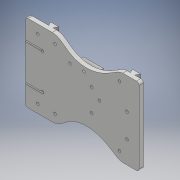
# Autodesk Inventor part: one_part_body_V2
Saved by Autodesk Inventor 2017 (Build 210142000, 142)
## iProperties
Created: 2017-05-19
Part Number: one_part_body_V2
Material: Generic
Document SubType Name: Modeling
Designer: Andi
Density: 1 g/cm^3
Appearance: Default
Author: Andi
Autodesk Inventor part; units mm, degrees
ref_plane "YZ Plane" through (0, 0, 0) normal (1, 0, 0) x (0, 1, 0)
ref_plane "XZ Plane" through (0, 0, 0) normal (0, 1, 0) x (-1, 0, 0)
ref_plane "XY Plane" through (0, 0, 0) normal (0, 0, 1) x (1, 0, 0)
sketch "Sketch1" plane through (0, 0, 0) normal (0, 1, 0) x (-1, 0, 0)
  line L0 (0, 90) -> (-132, 90)
  line L1 (-132, 90) -> (-132, 0)
  line L2 (-132, 0) -> (0, 0)
  line L3 (0, 0) -> (0, 90)
  line L4 (0, 45) -> (-132, 45)
  line L5 (0, 65.5) -> (-20, 65.5)
  line L6 (-20, 65.5) -> (-20, 67)
  line L7 (-20, 67) -> (0, 67)
  line L8 (0, 67) -> (0, 65.5)
  line L9 (0, 23) -> (-20, 23)
  line L10 (-20, 23) -> (-20, 24.5)
  line L11 (-20, 24.5) -> (0, 24.5)
  line L12 (0, 24.5) -> (0, 23)
  circle A0 centre (-20, 65.5) radius 1.5
  circle A1 centre (-20, 24.5) radius 1.5
  dimension "d0" = 132
  dimension "d1" = 90
  dimension "d2" = 20
  dimension "d3" = 41
  dimension "d4" = 1.5
  dimension "d5" = 1.5
  constraints: 26 end point, 6 parallel, 3 coincident, 3 horizontal, 3 perpendicular, 3 point on line, 2 midpoint, 2 vertical alignment, 1 symmetric about line, 4 other
  measures "d0" distance of L2.end L1.end
  measures "d1" distance of L2.end L0.start
  measures "d2" distance of L6.end L7.end
  measures "d3" distance of L11.end L5.start
  measures "d4" distance of L5.end L6.end
  measures "d5" distance of L9.end L10.end
extrude "Extrusion1" add sketch "Sketch1" along normal blind 5 contours L3 L7 A0 L5 L4 L1 L0 | L4 L3 L11 A1 L9 L2 L1
sketch "Sketch2" plane through (0, 0, 90) normal (0, 0, 1) x (1, 0, 0)
  line L0 (0, 5) -> (132, 5) projected
  line L1 (22, 5) -> (19.75, 9.5)
  line L2 (19.75, 9.5) -> (29.25, 9.5)
  line L3 (29.25, 9.5) -> (27, 5)
  line L4 (24.5, 9.5) -> (24.5, 0)
  line L5 (132, 0) -> (0, 0) projected
  line L6 (72, 0) -> (72, 13)
  line L7 (132, 0) -> (132, 5) projected
  line L8 (122, 5) -> (124.25, 9.5)
  line L9 (124.25, 9.5) -> (114.75, 9.5)
  line L10 (114.75, 9.5) -> (117, 5)
  line L11 (117, 5) -> (122, 5)
  line L12 (132, 5) -> (0, 5) projected
  dimension "d8" = 9.5
  dimension "d10" = 22
  dimension "d11" = 5
  dimension "d15" = 4.5
  dimension "d90" = 60
  constraints: 18 end point, 4 point on line, 4 symmetric about line, 2 perpendicular, 1 collinear, 1 midpoint, 1 parallel, 1 vertical, 1 other
  measures "d8" distance of L1.end L2.end
  measures "d10" distance of L1.start L0.start
  measures "d11" distance of L3.end L1.start
  measures "d15" distance between parallel lines of L2 L0
  measures "d90" distance between parallel lines of L7 L6
extrude "Extrusion7" add sketch "Sketch2" against normal up to surface (90 mm away) contours L10 L9 L8 L0 | L0 L4 L2 L3 | L0 L1 L2 L4
sketch "Sketch3" plane through (132, 0, 90) normal (1, 0, 0) x (0, 0, -1)
  line L0 (0, 0) -> (90, 0) projected
  line L1 (0, 9.5) -> (90, 9.5) projected
  line L2 (90, 5) -> (0, 5) projected
  line L3 (22.5, 9.5) -> (67.5, 9.5)
  line L4 (67.5, 9.5) -> (67.5, 5)
  line L5 (67.5, 5) -> (22.5, 5)
  line L6 (22.5, 5) -> (22.5, 9.5)
  line L7 (0, 9.5) -> (0, 5) projected
  line L8 (90, 5) -> (90, 9.5) projected
  dimension "d93" = 45
  dimension "d94" = 22.5
  dimension "d95" = 22.5
  constraints: 8 end point, 2 parallel, 2 point on line, 1 horizontal, 1 perpendicular
  measures "d93" distance between parallel lines of L4 L6
  measures "d94" distance between parallel lines of L7 L6
  measures "d95" distance between parallel lines of L8 L4
extrude "Extrusion3" cut sketch "Sketch3" against normal blind 120 contours L1 L4 L2 L6
sketch "Sketch4" plane through (0, 5, 0) normal (0, 1, 0) x (1, 0, 0)
  line L0 (50, -27) -> (70, -27)
  line L1 (70, -27) -> (70, -63)
  line L2 (70, -63) -> (50, -63)
  line L3 (50, -63) -> (50, -66)
  line L4 (50, -66) -> (73, -66)
  line L5 (73, -66) -> (73, -24)
  line L6 (73, -24) -> (50, -24)
  line L7 (50, -24) -> (50, -27)
  line L8 (132, -90) -> (132, 0) projected
  line L9 (132, -45) -> (0, -45)
  line L10 (0, -24.5) -> (0, -65.5) projected
  point P0 (0, 0)
  dimension "d25" = 3
  dimension "d26" = 70
  dimension "d27" = 3
  dimension "d28" = 20
  dimension "d29" = 36
  constraints: 18 end point, 7 perpendicular, 2 horizontal, 1 midpoint, 1 point on line, 2 other
  measures "d25" distance of L6.end L0.start
  measures "d26" distance between parallel lines of L10 L1
  measures "d27" distance between parallel lines of L1 L5
  measures "d28" distance of L0.start L0.end
  measures "d29" distance of L0.end L1.end
extrude "Extrusion4" add sketch "Sketch4" along normal blind 11
sketch "Sketch5" plane through (0, 16, 0) normal (0, 1, 0) x (1, 0, 0)
  line L0 (73, -24) -> (50, -24) projected
  line L1 (50, -63) -> (50, -66) projected
  line L2 (73, -24) -> (50, -24)
  line L3 (50, -24) -> (50, -66)
  line L4 (50, -66) -> (73, -66)
  line L5 (73, -66) -> (73, -24)
  point P0 (0, 0)
  constraints: 8 end point, 2 parallel, 1 horizontal, 1 perpendicular
extrude "Extrusion5" add sketch "Sketch5" along normal blind 2
sketch "Sketch6" plane through (0, 0, 0) normal (0, -1, 0) x (1, 0, 0)
  line L0 (67.1453, 53) -> (87.1453, 53)
  line L1 (87.1453, 53) -> (87.1453, 37)
  line L2 (87.1453, 37) -> (67.1453, 37)
  line L3 (67.1453, 37) -> (67.1453, 53)
  line L4 (0, 90) -> (132, 90) projected
  line L5 (0, 24.5) -> (0, 65.5) projected
  line L6 (0, 45) -> (132, 45)
  line L7 (132, 90) -> (132, 0) projected
  line L8 (132, 0) -> (0, 0) projected
  line L9 (77.1453, 90) -> (77.1453, 0)
  line L10 (120, 85) -> (120, 62.5) projected
  line L11 (34, 85) -> (34, 62.5) projected
  line L12 (77.1453, 37) -> (77.1453, 32)
  line L13 (77.1453, 53) -> (77.1453, 58)
  line L14 (87.1453, 49) -> (86.1453, 49)
  dimension "d34" = 20
  dimension "d35" = 16
  dimension "d41" = 5
  dimension "d42" = 5
  dimension "d84" = 4
  dimension "d86" = 43.1454
  dimension "d88" = 43.1454
  dimension "d117" = 9
  constraints: 18 end point, 6 point on line, 4 midpoint, 2 parallel, 2 perpendicular, 1 horizontal, 4 other
  measures "d34" distance of L1.end L2.end
  measures "d35" distance of L0.end L1.end
  measures "d41" distance of L12.start L12.end
  measures "d42" distance of L13.start L13.end
  measures "d84" distance between parallel lines of L14 L0
  measures "d86" distance of L10.start L9.start
  measures "d88" distance from line of L9 L11.start
  measures "d117" distance from line of L9 L14.end
hole "Hole1" at (77.1453, 0, 32) at (86.1453, 0, 49) at (77.1453, 0, 58) direction (0, 1, 0) diameter 3 depth 8 tip angle 118
sketch "Sketch7" plane through (0, 0, 0) normal (0, -1, 0) x (1, 0, 0)
  line L0 (152, 71.65) -> (52, 71.65)
  line L1 (52, 71.65) -> (52, 18.35)
  line L2 (52, 18.35) -> (152, 18.35)
  line L3 (152, 18.35) -> (152, 71.65)
  line L4 (132, 90) -> (132, 0) projected
  line L5 (132, 45) -> (0, 45)
  line L6 (0, 24.5) -> (0, 65.5) projected
  line L7 (152, 25.95) -> (118.1, 25.95)
  line L8 (152, 53.85) -> (118.1, 53.85)
  line L9 (52, 69.15) -> (68, 69.15)
  line L10 (50, 66) -> (73, 66) projected
  point P0 (0, 0)
  dimension "d52" = 53.3
  dimension "d53" = 100
  dimension "d54" = 20
  dimension "d55" = 66.1
  dimension "d56" = 7.6
  dimension "d57" = 33.9
  dimension "d58" = 27.9
  dimension "d81" = 50.1
  dimension "d82" = 2.5
  dimension "d83" = 16
  constraints: 16 end point, 3 parallel, 3 point on line, 2 horizontal, 2 midpoint, 2 perpendicular, 1 other
  measures "d52" distance of L2.end L0.start
  measures "d53" distance of L0.start L0.end
  measures "d54" distance between parallel lines of L4 L3
  measures "d55" distance from line of L1 L7.end
  measures "d56" distance from line of L2 L7.end
  measures "d57" distance of L8.start L8.end
  measures "d58" distance between parallel lines of L7 L8
  measures "d81" horizontal distance of L8.end L9.end
  measures "d82" distance between parallel lines of L9 L0
  measures "d83" distance of L9.start L9.end
hole "Hole2" at (118.1, 0, 25.95) at (118.1, 0, 53.85) at (68, 0, 69.15) at (52, 0, 69.15) direction (0, 1, 0) diameter 3 depth 8 tip angle 118
chamfer "Chamfer1" distance 0.5 angle 45 6 edges at (61.5, 18, 24) (73, 18, 45) (61.5, 18, 66) (60, 16, 27) (70, 16, 45) (60, 16, 63)
fillet "Fillet1" radius 3 4 edges at (0, 2.5, 0) (0, 2.5, 90) (132, 2.5, 90) (132, 2.5, 0)
sketch "Sketch10" plane through (0, 0, 0) normal (0, -1, 0) x (1, 0, 0)
  line L0 (29.25, 90) -> (19.75, 90) projected
  line L1 (24.5, 0) -> (24.5, 90)
  line L2 (19.75, 90) -> (19.75, 67.5) projected
  line L3 (114.75, 90) -> (124.25, 90) projected
  line L4 (119.5, 90) -> (119.5, 0)
  line L5 (129, 0) -> (3, 0) projected
  line L6 (0, 80) -> (132, 80)
  line L7 (132, 87) -> (132, 3) projected
  line L8 (0, 10) -> (132, 10)
  line L9 (3, 90) -> (129, 90) projected
  line L10 (24.5, 80) -> (14.5, 80)
  line L11 (24.5, 80) -> (34.5, 80)
  line L12 (24.5, 10) -> (14.5, 10)
  line L13 (24.5, 10) -> (34.5, 10)
  line L14 (119.5, 10) -> (109.5, 10)
  line L15 (119.5, 80) -> (109.5, 80)
  point P0 (0, 0)
  dimension "d100" = 10
  dimension "d101" = 10
  dimension "d102" = 10
  dimension "d103" = 10
  dimension "d104" = 10
  dimension "d105" = 10
  dimension "d106" = 10
  dimension "d107" = 10
  constraints: 20 end point, 17 point on line, 2 midpoint, 2 parallel, 1 horizontal, 1 vertical
  measures "d100" distance between parallel lines of L6 L9
  measures "d101" distance between parallel lines of L5 L8
  measures "d102" distance of L10.start L10.end
  measures "d103" distance of L10.start L11.end
  measures "d104" distance of L12.start L12.end
  measures "d105" distance of L12.start L13.end
  measures "d106" distance of L14.start L14.end
  measures "d107" distance of L15.start L15.end
hole "Hole3" at (14.5, 0, 80) at (34.5, 0, 80) at (14.5, 0, 10) at (34.5, 0, 10) at (109.5, 0, 80) at (109.5, 0, 10) direction (0, 1, 0) diameter 3 depth 8 tip angle 118
sketch "Sketch11" plane through (0, 0, 0) normal (0, -1, 0) x (1, 0, 0)
  line L0 (129, 0) -> (3, 0) projected
  line L1 (31.1108, 0) -> (43.1108, 0) construction
  line L2 (43.1108, 0) -> (49, 21) construction
  line L3 (49, 21) -> (90.4829, 21) construction
  line L4 (90.4829, 21) -> (105.1108, 0) construction
  line L5 (105.1108, 0) -> (113.1108, 0) construction
  spline S0 degree 4 poles (31.1108, 0) (43.1108, 0) (49, 21) (90.4829, 21) (105.1108, 0) (113.1108, 0) knots 1 1 1 1 1 2 3 3 3 3 3
  line L6 (132, 87) -> (132, 3) projected
  line L7 (132, 45) -> (0, 45)
  line L8 (0, 24.5) -> (0, 65.5) projected
  line L9 (31.1108, 90) -> (43.1108, 90) construction
  line L10 (43.1108, 90) -> (49, 69) construction
  line L11 (49, 69) -> (90.4829, 69) construction
  line L12 (90.4829, 69) -> (105.1108, 90) construction
  line L13 (105.1108, 90) -> (113.1108, 90) construction
  spline S1 degree 4 poles (31.1108, 90) (43.1108, 90) (49, 69) (90.4829, 69) (105.1108, 90) (113.1108, 90) knots 1 1 1 1 1 2 3 3 3 3 3
  line L14 (3, 90) -> (129, 90) projected
  line L15 (27, 90) -> (117, 90) projected
  line L16 (31.1108, 90) -> (113.1108, 90)
  point P0 (0, 0)
  constraints: 6 symmetric about line, 5 point on line, 4 end point, 2 midpoint, 1 collinear, 1 horizontal, 6 other
extrude "Extrusion8" cut sketch "Sketch11" against normal blind 10
equation "\"d5\" = d4"
body "Solid1"
